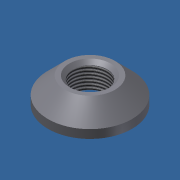
# Autodesk Inventor part: LUVA(24)
Saved by Autodesk Inventor 2012 SP1 (Build 160190100, 190)
## iProperties
Created: 2012-07-24
Part Number: LUVA(24)
Material: Carbon Steel
Document SubType Name: Modeling
Designer: bruno.silveira
Mass: 227.178 g
Surface Area: 61.8148 cm^2
Volume: 28.8663 cm^3
Density: 7.87 g/cm^3
Author: bruno.silveira
Autodesk Inventor part; units mm, degrees
ref_plane "YZ Plane" through (0, 0, 0) normal (1, 0, 0) x (0, 1, 0)
ref_plane "XZ Plane" through (0, 0, 0) normal (0, 1, 0) x (-1, 0, 0)
ref_plane "XY Plane" through (0, 0, 0) normal (0, 0, 1) x (1, 0, 0)
sketch "Sketch1" plane through (0, 0, 0) normal (0, 0, 1) x (1, 0, 0)
  circle A0 centre (0, 0) radius 24.75
  dimension "d0" = 49.5
  constraints: 1 centre point, 1 coincident
  measures "d0" diameter of A0
extrude "Extrusion1" add sketch "Sketch1" along normal blind 15
sketch "Sketch2" plane through (0, 0, 15) normal (0, 0, 1) x (1, 0, 0)
  circle A0 centre (0, 0) radius 24.75 projected
hole "Hole1" at (0, 0, 15) direction (0, 0, -1) diameter 20.269 depth 15 tip angle 118 thread size "7/8-14 UNF" class "2B" standard "ANSI Unified Screw Threads"
chamfer "Chamfer1" distance 10 angle 45 1 edges at (-24.75, 0, 15)
chamfer "Chamfer2" distance 2 angle 45 1 edges at (0, 10.1345, 15)
chamfer "Chamfer3" distance 0.5 angle 45 1 edges at (0, 10.1345, 0)
body "Solid1"
